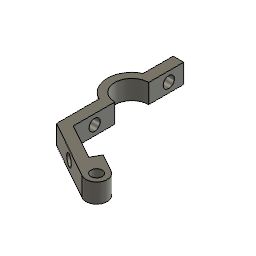
Trumpet+Clamp+1+Main (Autodesk Fusion 360 design; units mm, degrees)
Autodesk Fusion 360 part; units mm, degrees
sketch "Sketch1" plane through (0, 0, 0) normal (0, 1, 0) x (1, 0, 0)
  circle A0 centre (0, 0) radius 6.755
  circle A1 centre (0, 0) radius 9.755
  line L0 (0, 0) -> (-9.755, 0) construction
  line L1 (0, 0) -> (9.755, 0) construction
  line L2 (-4.25, -25.7687) -> (18.9274, -38.7154)
  line L3 (4.25, -20.7805) -> (23.0726, -31.2946)
  circle A2 centre (21, -35.005) radius 4.25
  line L4 (21, -35.005) -> (18.9274, -38.7154) construction
  line L5 (21, -35.005) -> (23.0726, -31.2946) construction
  circle A3 centre (21, -35.005) radius 2.25
  line L6 (-4.25, -25.7687) -> (-4.25, -8.7805)
  line L7 (4.25, -20.7805) -> (4.25, -8.7805)
  line L8 (0, 0) -> (0, -20.7805) construction
  line L9 (4.25, -20.7805) -> (-4.25, -20.7805) construction
  line L10 (-4.25, 8.7805) -> (-4.25, 20.7805)
  line L11 (-4.25, 20.7805) -> (4.25, 20.7805)
  line L12 (4.25, 20.7805) -> (4.25, 8.7805)
  line L13 (-4.25, 8.7805) -> (-4.25, -8.7805) construction
  line L14 (4.25, -8.7805) -> (4.25, 8.7805) construction
  line L15 (21, -35.005) -> (21, -39.255) construction
  point P0 (0, -9.755)
  dimension "d1" = 13.51
  dimension "d3" = 4.5
  dimension "d4" = 8.5
  dimension "d5" = 21
  dimension "d19" = 8.5
  dimension "d22" = 19.51
  dimension "d27" = 12
  dimension "d28" = 12
  dimension "d32" = 29.5
  constraint coincident A0.centre A1.centre
  constraint concentric A0 A1
  constraint coincident A1 L0.end
  constraint horizontal L0
  constraint coincident A1 L1.end
  constraint parallel L0 L1
  constraint coincident A2.centre L4.start
  constraint coincident A2 L2.end
  constraint coincident A2 L3.end
  constraint parallel L4 L5
  constraint coincident L2.end L4.end
  constraint coincident L3.end L5.end
  constraint coincident A1 L6.end
  constraint coincident A1 L7.end
  constraint parallel L2 L3
  constraint vertical L6
  constraint vertical L7
  constraint vertical L8
  constraint tangent L3 A2
  constraint coincident L6 L9.end
  constraint perpendicular L6 L9
  constraint midpoint L8.end L9
  constraint coincident A1 L10.start
  constraint vertical L10
  constraint perpendicular L10 L11
  constraint coincident A1 L12.end
  constraint perpendicular L11 L12
  constraint vertical L13
  constraint vertical L14
  constraint coincident A2 L15.end
  constraint vertical L15
  constraint coincident A1 P0
  constraint coincident L8 P0
  measures "d1" diameter of A0
  measures "d3" diameter of A3
  measures "d4" diameter of A2
  measures "d5" horizontal distance of A0.centre A2.centre
  measures "d19" distance of L6 L7
  measures "d22" diameter of A1
  measures "d27" distance of L3.start L7.end
  measures "d28" distance of L11.end L12.end
  measures "d32" vertical distance of L15.end P0
extrude "Extrude1" add sketch "Sketch1" along normal blind 7.7
sketch "Sketch2" plane through (-7.8365, 0, 14.0291) normal (0.487666, 0, -0.87303) x (-0.87303, 0, -0.487666)
  line L0 (-35.4044, 0) -> (-13.8443, 0)
  line L1 (-13.8443, 0) -> (-13.8443, 7.7)
  line L2 (-13.8443, 7.7) -> (-35.4044, 7.7)
  line L3 (-35.4044, 7.7) -> (-35.4044, 0)
  line L4 (-13.8443, 3.85) -> (-35.4044, 3.85) construction
  circle A0 centre (-21.8443, 3.85) radius 2.25
  dimension "d29" = 8
  dimension "d30" = 4.5
  constraint midpoint L1 L4.start
  constraint midpoint L3 L4.end
  constraint coincident L4 A0.centre
  measures "d29" distance of L4.start A0.centre
  measures "d30" diameter of A0
extrude "Extrude2" cut sketch "Sketch2" against normal up to surface (8.5 mm away) contours A0
sketch "Sketch3" plane through (4.25, 0, 0) normal (1, 0, 0) x (0, 0, -1)
  line L0 (-20.7805, 0) -> (-8.7805, 0)
  line L1 (-8.7805, 0) -> (-8.7805, 7.7)
  line L2 (-8.7805, 7.7) -> (-20.7805, 7.7)
  line L3 (-20.7805, 7.7) -> (-20.7805, 0)
  line L4 (-8.7805, 3.85) -> (-20.7805, 3.85) construction
  circle A0 centre (-14.7805, 3.85) radius 2.25
  line L5 (8.7805, 0) -> (20.7805, 0)
  line L6 (20.7805, 0) -> (20.7805, 7.7)
  line L7 (20.7805, 7.7) -> (8.7805, 7.7)
  line L8 (8.7805, 7.7) -> (8.7805, 0)
  line L9 (8.7805, 3.85) -> (20.7805, 3.85) construction
  circle A1 centre (14.7805, 3.85) radius 2.25
  dimension "d16" = 4.5
  constraint midpoint L1 L4.start
  constraint midpoint L3 L4.end
  constraint midpoint L4 A0.centre
  constraint midpoint L8 L9.start
  constraint midpoint L6 L9.end
  constraint midpoint L9 A1.centre
  constraint equal A0 A1
  measures "d16" diameter of A0
extrude "Extrude3" cut sketch "Sketch3" against normal up to surface (8.5 mm away) contours A0 | A1
sketch "Sketch4" plane through (0, 0, 0) normal (1, 0, 0) x (0, 0, -1)
  line L0 (-20.7805, 0) -> (-8.7805, 0) construction
  line L1 (-8.7805, 0) -> (-8.7805, 7.7) construction
  line L2 (-8.7805, 7.7) -> (-20.7805, 7.7) construction
  line L3 (-20.7805, 7.7) -> (-20.7805, 0) construction
  line L4 (8.7805, 0) -> (-8.7805, 0) construction
  line L5 (-8.7805, 0) -> (-8.7805, 7.7) construction
  line L6 (8.7805, 7.7) -> (-8.7805, 7.7) construction
  line L7 (-8.7805, 7.7) -> (-8.7805, 0) construction
  line L8 (-8.7805, 0) -> (-25.7687, 0) construction
  line L9 (-25.7687, 0) -> (-25.7687, 7.7) construction
  line L10 (-25.7687, 7.7) -> (-8.7805, 7.7) construction
  line L11 (-8.7805, 7.7) -> (-8.7805, 0) construction
  line L12 (8.7805, 0) -> (-23.2746, 0)
  line L13 (-23.2746, 0) -> (-23.2746, 7.7)
  line L14 (-23.2746, 7.7) -> (8.7805, 7.7)
  line L15 (8.7805, 7.7) -> (8.7805, 0)
  line L16 (-25.7687, 7.7) -> (-20.7805, 7.7) construction
  line L17 (8.7805, 7.7) -> (8.7805, 0)
  line L18 (8.7805, 0) -> (-8.7805, 0)
  line L19 (8.7805, 0) -> (8.7805, 7.7)
  line L20 (8.7805, 7.7) -> (-8.7805, 7.7)
  circle A0 centre (14.7805, 3.85) radius 2.25
  line L21 (8.7805, 0) -> (20.7805, 0)
  line L22 (20.7805, 0) -> (20.7805, 7.7)
  line L23 (20.7805, 7.7) -> (8.7805, 7.7)
  line L24 (8.7805, 7.7) -> (8.7805, 0)
  circle A1 centre (-14.7805, 3.85) radius 2.25
  circle A2 centre (-14.7805, 3.85) radius 2.25
  constraint horizontal L12
  constraint vertical L13
  constraint horizontal L14
  constraint vertical L15
  constraint coincident L10 L13.end
  constraint coincident L4.start L12.start
  constraint coincident L9.end L10.start
  constraint coincident L2.end L3.start
  constraint midpoint L13.end L16
extrude "Extrude4" cut sketch "Sketch4" along normal blind 14 contours L12 L13 L14 L15 L17 L18 L19 L20 L24 | L15 L17 L19 L21 L22 L23 L24 | A1 A2
ref_plane "WorkPlane1" through (9.4113, 3.85, 28.5317) normal (-0.487666, 0, 0.87303) x (0.87303, 0, 0.487666)
sketch "Sketch5" plane through (-9.9091, 0, 17.7395) normal (-0.487666, 0, 0.87303) x (0.87303, 0, 0.487666)
  line L0 (18.9587, 0) -> (11.3502, 0) construction
  line L1 (11.3502, 7.7) -> (18.9587, 7.7) construction
  line L2 (18.9587, 7.7) -> (35.4044, 7.7) construction
  line L3 (35.4044, 7.7) -> (35.4044, 0) construction
  line L4 (35.4044, 0) -> (18.9587, 0) construction
  line L5 (11.3502, 0) -> (27.1815, 0)
  line L6 (27.1815, 0) -> (27.1815, 7.7)
  line L7 (27.1815, 7.7) -> (11.3502, 7.7)
  line L8 (11.3502, 7.7) -> (11.3502, 0)
  line L9 (18.9587, 7.7) -> (18.9587, 0)
  line L10 (11.3502, 0) -> (11.3502, 7.7)
  line L11 (18.9587, 0) -> (18.9587, 7.7)
  circle A0 centre (21.8443, 3.85) radius 2.25
  point P0 (27.1815, 7.7)
  constraint horizontal L5
  constraint vertical L6
  constraint horizontal L7
  constraint vertical L8
  constraint coincident L2 P0
  constraint coincident L0.end L5.start
  constraint midpoint L2 P0
  constraint coincident L6 P0
extrude "Extrude5" cut sketch "Sketch5" against normal blind 15.688 contours L5 L7 L8 L9 L10 L11 | L5 L6 L7 L9 L11 | A0
equation "d19 = d4"
equation "d22 = d1 + 6 mm"
